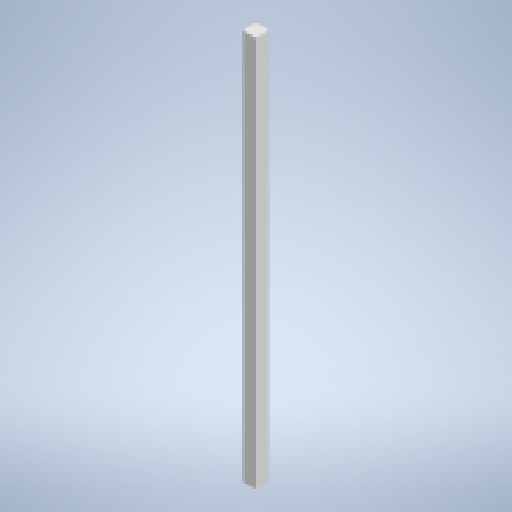
# Autodesk Inventor part: drive_shaft
Saved by Autodesk Inventor 2023 (Build 270158000, 158)
## iProperties
Created: 2023-11-28
Part Number: drive_shaft
Material: Generic
Document SubType Name: Modeling
Designer: Nate
Density: 1 g/cm^3
Appearance: Default
Author: Nate
Autodesk Inventor part; units mm, degrees
ref_plane "YZ Plane" through (0, 0, 0) normal (1, 0, 0) x (0, 1, 0)
ref_plane "XZ Plane" through (0, 0, 0) normal (0, 1, 0) x (-1, 0, 0)
ref_plane "XY Plane" through (0, 0, 0) normal (0, 0, 1) x (1, 0, 0)
sketch "Sketch1" plane through (0, 0, 0) normal (0, 0, 1) x (1, 0, 0)
  line L0 (0, 0) -> (4.7625, 0)
  line L1 (4.7625, 0) -> (4.7625, -139.7)
  line L2 (4.7625, -139.7) -> (0, -139.7)
  line L3 (0, -139.7) -> (0, 0)
  point P0 (2.3812, 0)
  point P1 (2.3813, -139.7)
  dimension "d1" = 139.7
  dimension "d2" = 4.7625
  constraints: 8 end point, 2 midpoint, 2 parallel, 1 horizontal, 1 perpendicular
  measures "d1" distance from line of point (2.381, -139.7) L0
  measures "d2" distance between parallel lines of L1 L3
extrude "Extrusion1" add sketch "Sketch1" along normal blind 4.7625
body "Solid1"
